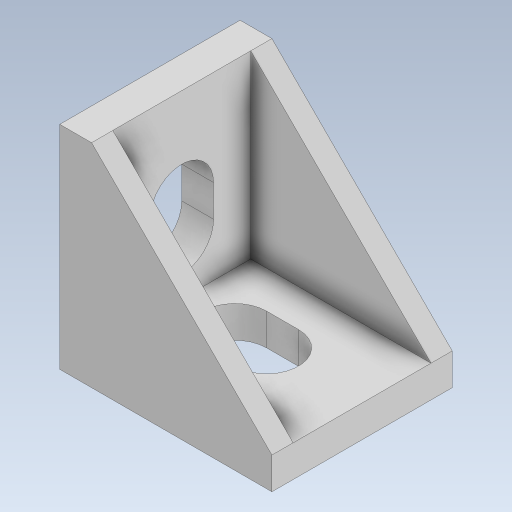
# Autodesk Inventor part: 20x20 90 Gusset
Saved by Autodesk Inventor 2023 (Build 270158000, 158)
## iProperties
Created: 2022-07-10
Part Number: 20x20 90 Gusset
Material: Generic
Document SubType Name: Modeling
Designer: Dave
Density: 1 g/cm^3
Appearance: Default
Author: Dave
Autodesk Inventor part; units mm, degrees
ref_plane "YZ Plane" through (0, 0, 0) normal (1, 0, 0) x (0, 1, 0)
ref_plane "XZ Plane" through (0, 0, 0) normal (0, 1, 0) x (-1, 0, 0)
ref_plane "XY Plane" through (0, 0, 0) normal (0, 0, 1) x (1, 0, 0)
sketch "Sketch2" plane through (0, 0, 0) normal (0, 0, 1) x (1, 0, 0)
  line L0 (3, 20) -> (0, 20)
  line L1 (0, 20) -> (0, 0)
  line L2 (0, 0) -> (20, 0)
  line L3 (20, 0) -> (20, 3)
  line L4 (20, 3) -> (3, 3)
  line L5 (3, 3) -> (3, 20)
  dimension "d0" = 20
  dimension "d1" = 3
  constraints: 12 end point, 6 perpendicular, 1 horizontal, 1 vertical
  measures "d0" distance of L0.end L1.end
  measures "d1" distance of L0.start L0.end
extrude "Extrusion1" add sketch "Sketch2" along normal blind 17
ref_plane "Work Plane1" through (3, 20, 0) normal (0.7071068, 0.7071068, 0) x (0, 0, 1)
sketch "Sketch3" plane through (3, 20, 0) normal (0.7071068, 0.7071068, 0) x (0, 0, 1)
  line L0 (0, 24.0416) -> (17, 24.0416) projected
  line L1 (17, 0) -> (15, 0)
  line L2 (15, 0) -> (15, 24.0416)
  line L3 (15, 24.0416) -> (17, 24.0416)
  line L4 (17, 24.0416) -> (17, 0)
  line L5 (0, 24.0416) -> (2, 24.0416)
  line L6 (2, 24.0416) -> (2, 0)
  line L7 (2, 0) -> (0, 0)
  line L8 (0, 0) -> (0, 24.0416)
  point P0 (0, 12.0208)
  dimension "d4" = 2
  dimension "d5" = 2
  constraints: 16 end point, 4 parallel, 2 horizontal, 2 perpendicular, 2 point on line
  measures "d4" distance of L6.end L7.end
  measures "d5" distance of L1.start L1.end
extrude "Extrusion2" add sketch "Sketch3" against normal up to next
sketch "Sketch4" plane through (3, 3, 2) normal (0, 1, 0) x (1, 0, 0)
  arc A0 (5, -3.5) -> (5, -9.5) centre (5, -6.5) ccw
  arc A1 (8, -9.5) -> (8, -3.5) centre (8, -6.5) ccw
  line L0 (8, -3.5) -> (5, -3.5)
  line L1 (8, -9.5) -> (5, -9.5)
  line L2 (-3, 2) -> (-3, -15) projected
  point P0 (-3, -6.5)
  point P1 (-3, -6.5)
  dimension "d8" = 6
  dimension "d9" = 6
  dimension "d10" = 3
  dimension "d11" = 8
  constraints: 4 end point, 4 point on circle, 4 tangent, 2 centre point, 2 horizontal alignment, 2 midpoint
  measures "d8" diameter of A0
  measures "d9" diameter of A1
  measures "d10" distance of L0.end L0.start
  measures "d11" distance of point (-3, -6.5) A0.centre
extrude "Extrusion3" cut sketch "Sketch4" against normal blind 6
pattern_circular "Circular Pattern2" count 2 over 90 about axis through (0, 0, 0) along (0, 0, 1) of "Extrusion3"
equation "\"d5\" = d4"
equation "\"d9\" = d8"
body "Solid1"
